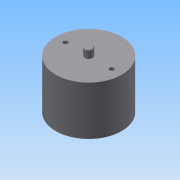
# Autodesk Inventor part: Tunel_Motor
Saved by Autodesk Inventor 2016 (Build 200138000, 138)
## iProperties
Created: 2014-11-24
Part Number: Tunel_Motor
Material: Generisch
Document SubType Name: Modeling
Designer: Gero Hofmann
Density: 1 g/cm^3
Appearance: Vorgabe
Author: Gero Hofmann
Autodesk Inventor part; units mm, degrees
ref_plane "YZ Plane" through (0, 0, 0) normal (1, 0, 0) x (0, 1, 0)
ref_plane "XY Plane" through (0, 0, 0) normal (0, 0, 1) x (1, 0, 0)
sketch "Skizze1" plane through (0, 0, 0) normal (0, 0, 1) x (1, 0, 0)
  circle A0 centre (0, 0) radius 25
  dimension "d0" = 50
  constraints: 1 centre point, 1 coincident
  measures "d0" diameter of A0
extrude "Extrusion1" add sketch "Skizze1" along normal mid plane 37
sketch "Skizze2" plane through (0, 0, 18.5) normal (0, 0, 1) x (1, 0, 0)
  circle A0 centre (0, 0) radius 25 projected
  circle A1 centre (0, 0) radius 3
  dimension "d3" = 6
  constraints: 1 centre point, 1 coincident
  measures "d3" diameter of A1
extrude "Extrusion2" add sketch "Skizze2" along normal blind 6 contours A1
sketch "Skizze3" plane through (0, 0, -18.5) normal (0, 0, -1) x (-1, 0, 0)
  circle A0 centre (0, 0) radius 25 projected
  circle A1 centre (0, 0) radius 3
  dimension "d6" = 6
  constraints: 1 centre point, 1 coincident
  measures "d6" diameter of A1
extrude "Extrusion3" add sketch "Skizze3" along normal blind 15 contours A1
chamfer "Fase1" distance 0.5 angle 45 2 edges at (3, 0, -33.5) (-3, 0, 24.5)
sketch "Skizze4" plane through (0, 0, 18.5) normal (0, 0, 1) x (1, 0, 0)
  circle A0 centre (0, 0) radius 3 projected
  line L0 (-17.5, 0) -> (17.5, 0) construction
  dimension "d12" = 35
  constraints: 2 end point, 1 coincident, 1 horizontal, 1 midpoint
  measures "d12" distance of L0.start L0.end
hole "Bohrung1" at (-17.5, 0, 18.5) at (17.5, 0, 18.5) direction (0, 0, -1) diameter 3.242 depth 8 tip angle 118 thread size "M4x0.7" class "6H" standard "ISO Metric profile"
mirror "Spiegeln1" about plane through (0, 0, 0) normal (0, 0, 1) of "Bohrung1"
ref_plane "Arbeitsebene1" through (0, 25, 0) normal (0, 1, 0) x (-1, 0, 0)
sketch "Skizze5" plane through (0, 25, 0) normal (0, 1, 0) x (-1, 0, 0)
  line L0 (-25, -18.5) -> (25, -18.5) projected
  line L1 (25, 18.5) -> (-25, 18.5) projected
  circle A0 centre (0, 3.5) radius 2.5
  point P0 (0, 0)
  dimension "d20" = 15
  dimension "d21" = 5
  constraints: 1 centre point, 1 coincident
  measures "d20" distance from line of L1 point (0, 3.5)
  measures "d21" diameter of A0
extrude "Extrusion4" add sketch "Skizze5" against normal blind 2 and the other way blind 2
